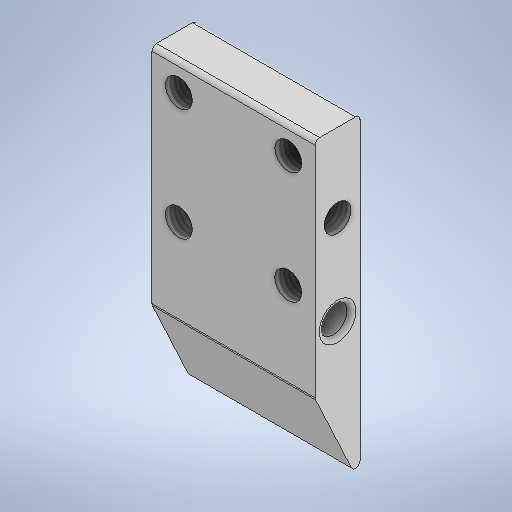
# Autodesk Inventor part: Pedal Support 1
Saved by Autodesk Inventor 2025.2 (Build 292293000, 293)
## iProperties
Created: 2025-03-16
Part Number: Pedal Support 1
Material: Generic
Document SubType Name: Modeling
Designer: eason
Density: 1 g/cm^3
Appearance: Default
Author: eason
Autodesk Inventor part; units mm, degrees
ref_plane "YZ Plane" through (0, 0, 0) normal (1, 0, 0) x (0, 1, 0)
ref_plane "XZ Plane" through (0, 0, 0) normal (0, 1, 0) x (-1, 0, 0)
ref_plane "XY Plane" through (0, 0, 0) normal (0, 0, 1) x (1, 0, 0)
sketch "Sketch1" plane through (0, 0, 0) normal (0, 0, 1) x (1, 0, 0)
  line L0 (-18.2, 27.5) -> (18.2, 27.5)
  line L1 (18.2, 27.5) -> (18.2, -27.5)
  line L2 (18.2, -27.5) -> (-18.2, -27.5)
  line L3 (-18.2, -27.5) -> (-18.2, 27.5)
  line L4 (0, -38.5) -> (0, 38.5) projected
  line L5 (-25.48, 0) -> (25.48, 0) projected
  circle A0 centre (-12.2, 21.5) radius 3
  circle A1 centre (-12.2, 21.5) radius 6 construction
  circle A2 centre (-12.2, -3.5) radius 3
  line L6 (-12.2, 27.5) -> (-12.2, -3.5) construction
  circle A3 centre (12.2, 21.5) radius 3
  circle A4 centre (12.2, -3.5) radius 3
  point P0 (0, 0)
  point P1 (0, 27.5)
  point P2 (-18.2, 0)
  dimension "d0" = 36.4
  dimension "d1" = 55
  dimension "d2" = 6
  dimension "d3" = 3
  dimension "d34" = 25
  constraints: 10 end point, 4 centre point, 3 point on line, 2 horizontal, 2 midpoint, 2 parallel, 2 perpendicular, 2 symmetric about line, 1 coincident, 1 equal radius, 1 vertical, 1 vertical alignment, 4 other
  measures "d0" distance between parallel lines of L1 L3
  measures "d1" distance of L0.end L1.end
  measures "d2" diameter of A0
  measures "d3" radius of A0
  measures "d34" distance of L6.end A0.centre
extrude "Extrusion1" add sketch "Sketch1" along normal blind 10
sketch "Sketch4" plane through (18.2, -27.5, 0) normal (1, 0, 0) x (0, 0, -1)
  circle A0 centre (-5, 17.5) radius 3 construction
  line L0 (-10, 55) -> (-10, 0) projected
  line L1 (-10, 27.5) -> (0, 27.5) construction
  line L2 (0, 55) -> (0, 0) projected
  circle A1 centre (-5, 37.5) radius 3
  line L3 (0, 0) -> (-10, 0) projected
  line L4 (-5, 0) -> (-5, 55) construction
  line L5 (0, 55) -> (-10, 55) projected
  circle A2 centre (-5, 17.5) radius 3.1
  dimension "d20" = 6
  dimension "d21" = 20
  dimension "d24" = 6.2
  constraints: 4 end point, 4 midpoint, 3 centre point, 1 coincident, 1 point on line, 1 symmetric about line, 1 other
  measures "d20" diameter of A0
  measures "d21" distance of A1.centre A0.centre
  measures "d24" diameter of A2
extrude "Extrusion4" cut sketch "Sketch4" against normal up to surface (36.4 mm away) contours A1 | A2
thread "Thread1" size "M6x1" class "6H" standard "ANSI Metric M Profile" full length
sketch "Sketch5" plane through (18.2, -27.5, 0) normal (1, 0, 0) x (0, 0, -1)
  line L0 (-10, 55) -> (-10, 0) projected
  line L1 (0, -16.4451) -> (0, 0)
  line L2 (0, 0) -> (0, 55) projected
  line L3 (0, 0) -> (-10, 0) projected
  line L4 (0, -16.4451) -> (-10, 5)
  point P0 (0, 27.5)
  point P1 (-7.6685, 0)
  dimension "d30" = 5
  dimension "d31" = 25
  constraints: 4 end point, 1 collinear, 1 parallel, 1 point on line
  measures "d30" distance of L0.end L4.end
  measures "d31" angle of L1 L4
extrude "Extrusion5" add sketch "Sketch5" against normal up to surface (36.4 mm away) contours L3 L1 L4
extrude "Extrusion6" cut sketch "Sketch5" against normal up to surface (36.4 mm away) contours L4 L3 L0
fillet "Fillet1" radius 1 5 edges at (0, 27.5, 0) (0, 27.5, 10) (0, -43.9451, 0) (18.2, -10, 8.1) (-18.2, -10, 8.1)
thread "Thread2" size "M6x1" class "6H" standard "ANSI Metric M Profile" full length
thread "Thread3" size "M6x1" class "6H" standard "ANSI Metric M Profile" full length
thread "Thread4" size "M6x1" class "6H" standard "ANSI Metric M Profile" full length
thread "Thread5" size "M6x1" class "6H" standard "ANSI Metric M Profile" full length
body "Solid1"
